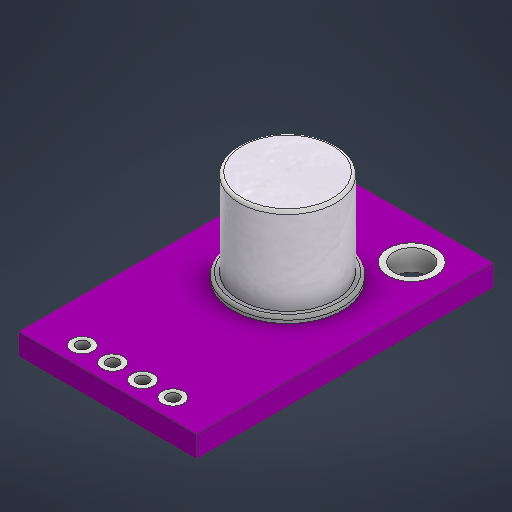
# Autodesk Inventor part: Gas_Sensorsipt
Saved by Autodesk Inventor 2026 (Build 300175000, 175)
## iProperties
Created: 2025-04-13
Part Number: Gas_Sensorsipt
Material: Generic
Document SubType Name: Modeling
Designer: ct_vi
Density: 1 g/cm^3
Appearance: Default
Author: ct_vi
Autodesk Inventor part; units mm, degrees
ref_plane "YZ Plane" through (0, 0, 0) normal (1, 0, 0) x (0, 1, 0)
ref_plane "XZ Plane" through (0, 0, 0) normal (0, 1, 0) x (-1, 0, 0)
ref_plane "XY Plane" through (0, 0, 0) normal (0, 0, 1) x (1, 0, 0)
sketch "Sketch1" plane through (0, 0, 0) normal (0, 1, 0) x (-1, 0, 0)
  line L0 (7.5, 12.1) -> (-7.5, 12.1)
  line L1 (-7.5, 12.1) -> (-7.5, -12.9)
  line L2 (-7.5, -12.9) -> (7.5, -12.9)
  line L3 (7.5, -12.9) -> (7.5, 12.1)
  circle A0 centre (0, -3.0541) radius 4.05
  circle A1 centre (0, -3.0541) radius 4.6
  circle A2 centre (4, -9.5) radius 1.5
  line L4 (7.5, -12.9) -> (4, -12.9)
  circle A3 centre (-4, -9.5) radius 1.5
  circle A4 centre (4, -9.5) radius 2
  circle A5 centre (-4, -9.5) radius 2
  line L5 (0, -3.0541) -> (7.5, -3.0541)
  line L6 (7.5, -3.0541) -> (7.5, -12.9)
  line L7 (7.5, -12.9) -> (0, -12.9)
  line L8 (0, -12.9) -> (0, -3.0541)
  line L9 (8.662, 14.258) -> (8.662, -14.1579) construction
  line L10 (8.662, -14.1579) -> (-25.9569, -14.1579) construction
  line L11 (-25.9569, -14.1579) -> (-25.9569, 14.258) construction
  line L12 (-25.9569, 14.258) -> (8.662, 14.258) construction
  line L13 (0, -3.0541) -> (0, 12.1)
  line L14 (0, 12.1) -> (0, 10.4)
  line L15 (0, 10.4) -> (1.27, 10.4)
  line L16 (1.27, 10.4) -> (3.81, 10.4)
  line L17 (0, 10.4) -> (-1.27, 10.4)
  line L18 (-1.27, 10.4) -> (-3.81, 10.4)
  circle A6 centre (1.27, 10.4) radius 0.5
  circle A7 centre (3.81, 10.4) radius 0.5
  circle A8 centre (3.81, 10.4) radius 0.9
  circle A9 centre (1.27, 10.4) radius 0.9
  circle A10 centre (-1.27, 10.4) radius 0.9
  circle A11 centre (-3.81, 10.4) radius 0.9
  circle A12 centre (-1.27, 10.4) radius 0.5
  circle A13 centre (-3.81, 10.4) radius 0.5
  point P0 (0, 0)
  dimension "d0" = 15
  dimension "d1" = 25
  dimension "d64" = 8.1
  dimension "d68" = 9.2
  dimension "d73" = 3
  dimension "d83" = 3
  dimension "d99" = 0.5
  dimension "d100" = 0.5
  dimension "d113" = 9.846
  dimension "d114" = 3.5
  dimension "d115" = 3.4
  dimension "d143" = 1.7
  dimension "d144" = 1.27
  dimension "d145" = 2.54
  dimension "d146" = 1.27
  dimension "d147" = 2.54
  dimension "d148" = 1
  dimension "d149" = 1
  dimension "d150" = 1.8
  dimension "d151" = 1.8
  dimension "d152" = 1.8
  dimension "d153" = 1.8
  dimension "d154" = 1
  dimension "d155" = 1
  constraints: 30 end point, 14 centre point, 9 coincident, 4 horizontal, 4 parallel, 3 perpendicular, 3 point on line, 1 midpoint, 2 other
  measures "d0" distance of L2.end L1.end
  measures "d1" distance of L1.end L0.end
  measures "d64" diameter of A0
  measures "d68" diameter of A1
  measures "d73" diameter of A2
  measures "d83" diameter of A3
  measures "d99" radial gap between concentric circles of A2 A4
  measures "d100" radial gap between concentric circles of A3 A5
  measures "d113" distance of L7.end L5.start
  measures "d114" distance from line of A2.centre L3
  measures "d115" distance from line of A2.centre L2
  measures "d143" distance of L13.end L14.end
  measures "d144" distance of L14.end L15.end
  measures "d145" distance of L15.end L16.end
  measures "d146" distance of L14.end L17.end
  measures "d147" distance of L17.end L18.end
  measures "d148" diameter of A6
  measures "d149" diameter of A7
  measures "d150" diameter of A8
  measures "d151" diameter of A9
  measures "d152" diameter of A10
  measures "d153" diameter of A11
  measures "d154" diameter of A12
  measures "d155" diameter of A13
extrude "Extrusion1" add sketch "Sketch1" against normal blind 1.8 contours L3 L5 A1 L13 L0 | L13 A1 L8 L2 L1 L0 | L3 L2 L8 A1 L5 | L5 A0 L13 A1 | A1 L8 A0 L5 | L13 A0 L8 A1 | L5 L13 A0 | A0 L8 L5 | L13 L8 A0 | A2 | A3 | A4 | A5 | A9 L16 A6 L15 | L15 A6 L16 A9 | A6 L16 L15 | L15 L16 A6 | A10 L18 A12 L17 | L17 A12 L18 A10 | A12 L18 L17 | L17 L18 A12 | A7 | A8 | A11 | A13
extrude "Extrusion2" cut sketch "Sketch1" against normal through all contours A2 | A3 | A4 | A5
extrude "Extrusion3" add sketch "Sketch1" against normal blind 1.8 contours A4 | A5
extrude "Extrusion4" add sketch "Sketch1" along normal blind 7.8 contours L5 L13 A0 | A0 L8 L5 | L13 L8 A0
extrude "Extrusion5" add sketch "Sketch1" along normal blind 0.5 contours L5 A0 L13 A1 | A1 L8 A0 L5 | L13 A0 L8 A1
fillet "Fillet1" radius 0.25 1 edges at (4.05, 7.8, -3.0541)
fillet "Fillet2" radius 0.25 1 edges at (4.6, 0.5, -3.0541)
extrude "Extrusion6" cut sketch "Sketch1" against normal blind 10 contours A6 L16 L15 | L15 L16 A6 | A12 L18 L17 | L17 L18 A12 | A7 | A13
extrude "Extrusion7" cut sketch "Sketch1" against normal blind 10 contours A9 L16 A6 L15 | L15 A6 L16 A9 | A10 L18 A12 L17 | L17 A12 L18 A10 | A8 | A11
extrude "Extrusion8" add sketch "Sketch1" against normal up to surface (1.8 mm away) separate body contours A4 | A5 | A9 L16 A6 L15 | L15 A6 L16 A9 | A10 L18 A12 L17 | L17 A12 L18 A10 | A8 | A11
extrude "Extrusion9" cut sketch "Sketch1" against normal through all contours A4 | A5 bodies 1
body "Solid1"
body "Solid2"
